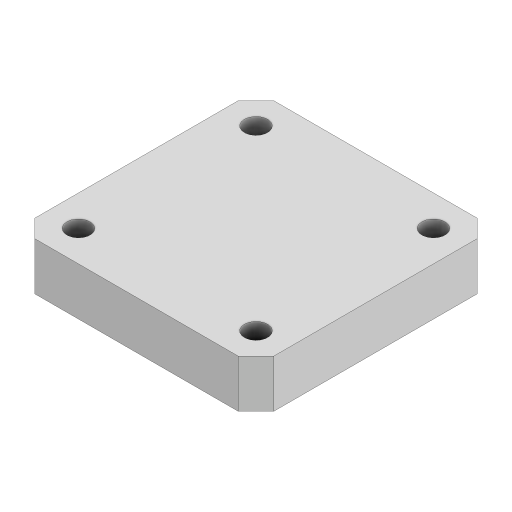
# Autodesk Inventor part: PCB_Spacer
Saved by Autodesk Inventor 2023 (Build 270158000, 158)
## iProperties
Created: 2026-05-12
Part Number: PCB_Spacer
Material: Generic
Document SubType Name: Modeling
Designer: ferrerx
Density: 1 g/cm^3
Appearance: Default
Author: ferrerx
Autodesk Inventor part; units mm, degrees
ref_plane "YZ Plane" through (0, 0, 0) normal (1, 0, 0) x (0, 1, 0)
ref_plane "XZ Plane" through (0, 0, 0) normal (0, 1, 0) x (-1, 0, 0)
ref_plane "XY Plane" through (0, 0, 0) normal (0, 0, 1) x (1, 0, 0)
sketch "Sketch1" plane through (0, 0, 0) normal (0, 1, 0) x (-1, 0, 0)
  line L0 (-17.5, 17.5) -> (17.5, 17.5)
  line L1 (17.5, 17.5) -> (17.5, -17.5)
  line L2 (17.5, -17.5) -> (-17.5, -17.5)
  line L3 (-17.5, -17.5) -> (-17.5, 17.5)
  line L4 (-17.5, 17.5) -> (17.5, -17.5) construction
  line L5 (17.5, 17.5) -> (-17.5, -17.5) construction
  line L6 (-13, -13) -> (13, -13) construction
  line L7 (13, -13) -> (13, 13) construction
  line L8 (13, 13) -> (-13, 13) construction
  line L9 (-13, 13) -> (-13, -13) construction
  line L10 (-13, -13) -> (13, 13) construction
  line L11 (13, -13) -> (-13, 13) construction
  circle A0 centre (13, 13) radius 1.7
  circle A1 centre (13, -13) radius 1.7
  circle A2 centre (-13, -13) radius 1.7
  circle A3 centre (-13, 13) radius 1.7
  point P0 (0, 0)
  dimension "d0" = 35
  dimension "d1" = 35
  dimension "d2" = 3.4
  dimension "d3" = 3.4
  dimension "d4" = 3.4
  dimension "d5" = 3.4
  dimension "d6" = 26
  dimension "d7" = 26
  constraints: 24 end point, 4 centre point, 4 coincident, 4 midpoint, 4 parallel, 2 horizontal, 2 perpendicular
  measures "d0" distance of L1.end L2.end
  measures "d1" distance of L0.end L1.end
  measures "d2" diameter of A1
  measures "d3" diameter of A0
  measures "d4" diameter of A3
  measures "d5" diameter of A2
  measures "d6" distance of L7.end L8.end
  measures "d7" distance of L6.end L7.end
extrude "Extrusion1" add sketch "Sketch1" along normal blind 7
chamfer "Chamfer1" distance 2.6 angle 45 4 edges at (17.5, 3.5, 17.5) (-17.5, 3.5, 17.5) (17.5, 3.5, -17.5) (-17.5, 3.5, -17.5)
shell "Shell2" thickness 2 removed faces 1 at (-3.9092, 0, 3.9576)
equation "\"d1\" = d0"
equation "\"d3\" = d2"
equation "\"d4\" = d2"
equation "\"d5\" = d2"
body "Solid1"
